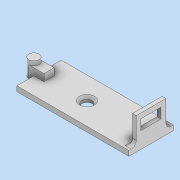
# Autodesk Inventor part: arduino_holder
Saved by Autodesk Inventor 2022 (Build 260153000, 153)
## iProperties
Created: 2022-08-22
Part Number: arduino_holder
Material: Générique
Document SubType Name: Modeling
Designer: andre
Density: 1 g/cm^3
Appearance: Par défaut
Author: andre
Autodesk Inventor part; units mm, degrees
ref_plane "YZ Plane" through (0, 0, 0) normal (1, 0, 0) x (0, 1, 0)
ref_plane "XZ Plane" through (0, 0, 0) normal (0, 1, 0) x (-1, 0, 0)
ref_plane "XY Plane" through (0, 0, 0) normal (0, 0, 1) x (1, 0, 0)
sketch "Esquisse1" plane through (0, 0, 0) normal (0, 1, 0) x (-1, 0, 0)
  line L0 (21.45, 8.8) -> (-21.45, 8.8)
  line L1 (-21.45, 8.8) -> (-21.45, -8.8)
  line L2 (-21.45, -8.8) -> (21.45, -8.8)
  line L3 (21.45, -8.8) -> (21.45, 8.8)
  line L4 (21.45, 8.8) -> (-21.45, -8.8) construction
  line L5 (-21.45, 8.8) -> (21.45, -8.8) construction
  point P0 (0, 0)
  dimension "d0" = 42.9
  dimension "d1" = 17.6
  constraints: 12 end point, 2 midpoint, 2 parallel, 1 horizontal, 1 perpendicular
  measures "d0" distance of L1.end L2.end
  measures "d1" distance of L2.end L0.start
extrude "Extrusion1" add sketch "Esquisse1" along normal blind 2
sketch "Esquisse2" plane through (21.45, 0, 8.8) normal (1, 0, 0) x (0, 0, -1)
  line L0 (4.6867, 10.5) -> (12.6867, 10.5)
  line L1 (12.6867, 10.5) -> (12.6867, 6.5)
  line L2 (12.6867, 6.5) -> (4.6867, 6.5)
  line L3 (4.6867, 6.5) -> (4.6867, 10.5)
  line L4 (4.6867, 10.5) -> (12.6867, 6.5) construction
  line L5 (12.6867, 10.5) -> (4.6867, 6.5) construction
  line L6 (2.9446, 12.5) -> (14.6867, 12.5)
  line L7 (14.6867, 12.5) -> (14.6867, 4.3203)
  line L8 (2.9446, 4.6719) -> (2.9446, 12.5)
  line L9 (2.9446, 12.5) -> (14.6867, 4.3203) construction
  line L10 (14.6867, 12.5) -> (2.9446, 4.6719) construction
  line L11 (0, 2) -> (17.6, 2) projected
  line L12 (2.9446, 4.6719) -> (2.9446, 0)
  line L13 (0, 0) -> (17.6, 0) projected
  line L14 (14.6867, 4.3203) -> (14.6867, 0)
  line L15 (2.9446, 0) -> (14.6867, 0)
  point P0 (8.8, 0)
  point P1 (8.6867, 8.5)
  point P2 (8.6867, 8.5)
  dimension "d4" = 4.5
  dimension "d6" = 2
  dimension "d7" = 8
  dimension "d8" = 4
  constraints: 28 end point, 3 midpoint, 3 parallel, 3 point on line, 2 horizontal, 2 perpendicular, 2 vertical, 1 collinear
  measures "d4" distance between parallel lines of L11 L2
  measures "d6" distance between parallel lines of L7 L1
  measures "d7" distance between parallel lines of L1 L3
  measures "d8" distance of L2.end L0.start
extrude "Extrusion2" add sketch "Esquisse2" along normal blind 1.5
sketch "Esquisse4" plane through (0, 2, 0) normal (0, 1, 0) x (1, 0, 0)
  line L0 (-21.45, 8.8) -> (-21.45, -8.8) projected
  point P0 (0, 0)
  point P1 (-2.45, 0)
  dimension "d18" = 19
  measures "d18" distance from line of L0 point (-2.45, 0)
hole "Perçage2" at (-2.45, 2, 0) direction (0, -1, 0) diameter 4 end through all countersink diameter 6 countersink angle 90
sketch "Esquisse5" plane through (21.45, 0, 8.8) normal (1, 0, 0) x (0, 0, -1)
  line L0 (0, 0) -> (2.9446, 0) projected
  line L1 (2.9446, 2) -> (14.6867, 2) projected
  line L2 (0, 0) -> (2.9446, 0)
  line L3 (2.9446, 0) -> (2.9446, 2)
  line L4 (2.9446, 2) -> (0, 2)
  line L5 (0, 2) -> (0, 0)
  line L6 (2.9446, 0) -> (14.6867, 0) projected
  line L7 (14.6867, 2) -> (17.6, 2) projected
  line L8 (14.6867, 0) -> (17.6, 0)
  line L9 (17.6, 0) -> (17.6, 2)
  line L10 (17.6, 2) -> (14.6867, 2)
  line L11 (14.6867, 2) -> (14.6867, 0)
  point P0 (8.8, 0)
  constraints: 16 end point, 4 parallel, 2 horizontal, 2 perpendicular
extrude "Extrusion3" add sketch "Esquisse5" along normal up to surface (1.5 mm away) contours L5 L4 L3 L0 | L11 L7 L9 L8
fillet "Congé1" radius 2 2 edges at (22.2, 2, 5.8554) (22.2, 2, -5.8867)
fillet "Congé2" radius 1 1 edges at (21.45, 2, -0.0157)
sketch "Esquisse6" plane through (0, 0, 0) normal (0, -1, 0) x (1, 0, 0)
  circle A0 centre (-23.45, 0) radius 2
  line L0 (-21.45, -8.8) -> (-21.45, 8.8) projected
  line L1 (-23.45, 2) -> (-17.45, 2)
  line L2 (-17.45, 2) -> (-17.45, -2)
  line L3 (-17.45, -2) -> (-23.45, -2)
  line L4 (0, 0) -> (4.0498, 0)
  dimension "d30" = 4
  dimension "d31" = 4
  constraints: 8 end point, 3 tangent, 2 horizontal, 2 point on circle, 1 centre point, 1 parallel, 1 perpendicular, 1 point on line
  measures "d30" diameter of A0
  measures "d31" distance between parallel lines of L2 L0
extrude "Extrusion4" add sketch "Esquisse6" against normal blind 4.8
sketch "Esquisse7" plane through (0, 4.8, 0) normal (0, 1, 0) x (1, 0, 0)
  circle A0 centre (-23.45, 0) radius 2
  arc A1 (-23.45, 2) -> (-23.45, -2) centre (-23.45, 0) ccw projected
  point P0 (0, 0)
  constraints: 1 centre point, 1 coincident, 1 concentric
extrude "Extrusion5" add sketch "Esquisse7" along normal blind 1.7
equation "\"d6\" = d5"
equation "\"d5\" = 2"
